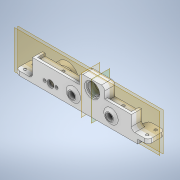
# Autodesk Inventor part: MotorBracket_v6.4
Saved by Autodesk Inventor 2022 (Build 260153000, 153)
## iProperties
Created: 2022-01-31
Part Number: MotorBracket_v6.4
Material: ABS プラスチック
Document SubType Name: Modeling
Designer: shiokaze
Density: 1.06 g/cm^3
Appearance: 滑らか - 白
Mass: 5.74152 g
Surface Area: 41.0545 cm^2
Volume: 5.41653 cm^3
Author: shiokaze
Autodesk Inventor part; units mm, degrees
ref_plane "YZ Plane" through (0, 0, 0) normal (1, 0, 0) x (0, 1, 0)
ref_plane "XZ Plane" through (0, 0, 0) normal (0, 1, 0) x (-1, 0, 0)
ref_plane "XY Plane" through (0, 0, 0) normal (0, 0, 1) x (1, 0, 0)
sketch "スケッチ2" plane through (0, 0, 0) normal (0, 0, 1) x (1, 0, 0)
  line L0 (-46.5, 9.7) -> (31.5, 9.7)
  line L1 (31.5, 9.7) -> (31.5, -9.7)
  line L2 (31.5, -9.7) -> (-46.5, -9.7)
  line L3 (-46.5, -9.7) -> (-46.5, 9.7)
  line L4 (-46.5, 9.7) -> (31.5, -9.7)
  line L5 (31.5, 9.7) -> (-46.5, -9.7)
  line L6 (-46.5, 9.7) -> (-8.95, 9.7)
  line L7 (-8.95, 9.7) -> (-8.95, -7.2)
  line L8 (-8.95, -7.2) -> (-46.5, -7.2)
  line L9 (-46.5, -7.2) -> (-46.5, 9.7)
  line L10 (31.5, 9.7) -> (5.95, 9.7)
  line L11 (5.95, 9.7) -> (5.95, -4.7)
  line L12 (5.95, -4.7) -> (31.5, -4.7)
  line L13 (31.5, -4.7) -> (31.5, 9.7)
  line L14 (-36.4485, -7.2) -> (-36.7, -7.2)
  line L15 (-36.7, -7.2) -> (-36.7, 3.5)
  line L16 (-36.7, 3.5) -> (-8.95, 3.5)
  line L17 (-8.95, 3.5) -> (-8.95, -0.3606)
  line L18 (5.95, -4.7) -> (21.7, -4.7)
  line L19 (21.7, -4.7) -> (21.7, 3.5)
  line L20 (21.7, 3.5) -> (5.95, 3.5)
  line L21 (5.95, 3.5) -> (5.95, -4.7)
  line L22 (31.5, -9.7) -> (25.5, -9.7)
  line L23 (25.5, -9.7) -> (25.5, -7.2)
  line L24 (25.5, -7.2) -> (31.5, -7.2)
  line L25 (31.5, -7.2) -> (31.5, -9.7)
  line L26 (-7.5, 0) -> (0, 0)
  point P0 (-7.5, 0)
  point P1 (5.95, 9.7)
  point P2 (-8.95, 9.7)
  point P3 (-8.95, 3.5)
  point P4 (-36.7, -7.2)
  point P5 (-46.5, -7.2)
  point P6 (31.5, -7.2)
  point P7 (31.5, -4.7)
  point P8 (21.7, -4.7)
  dimension "d0" = 78
  dimension "d1" = 19.4
  dimension "d15" = 37.55
  dimension "d16" = 2.5
  dimension "d17" = 25.55
  dimension "d18" = 6
  dimension "d19" = 2.5
  dimension "d20" = 9.8
  dimension "d21" = 9.8
  dimension "d26" = 7.5
  dimension "d188" = 10.7
  dimension "d241" = 5
  constraints: 54 end point, 12 parallel, 7 horizontal, 6 perpendicular, 3 collinear, 2 midpoint, 2 point on line, 1 coincident
  measures "d0" distance of L0.start L0.end
  measures "d1" distance of L0.end L1.end
  measures "d15" distance of L7.end L8.end
  measures "d16" distance between parallel lines of L2 L8
  measures "d17" distance of L12.end L11.end
  measures "d18" distance of L23.end L24.end
  measures "d19" distance of L22.end L23.end
  measures "d20" distance between parallel lines of L1 L19
  measures "d21" distance between parallel lines of L3 L15
  measures "d26" distance of L26.start L26.end
  measures "d188" distance between parallel lines of L16 L8
  measures "d241" distance between parallel lines of L18 L2
extrude "押し出し1" add sketch "スケッチ2" along normal blind 6 contours L0 L11 L5 L4 L7 | L8 L5 L3 | L16 L7 L4 | L4 L7 L5 L8 L15 L16 | L5 L8 L7 L4 L11 L12 L23 L2 | L4 L5 L7 | L20 L5 L11 | L5 L7 L8 | L5 L11 L4 | L1 L24 L23 L4 L12 | L20 L19 L12 L4 L11 L5 | L4 L12 L11
sketch "スケッチ8" plane through (0, 0, 6) normal (0, 0, 1) x (1, 0, 0)
  circle A0 centre (-1.5, 4.4354) radius 3.85 construction
  circle A1 centre (9.625, -3.3) radius 9.7 construction
  circle A2 centre (-12.625, -3.3) radius 9.7 construction
  circle A3 centre (-26.1025, -4.7) radius 3.85 construction
  line L0 (-46.5, -9.7) -> (25.5, -9.7) construction
  circle A4 centre (-12.625, -3.3) radius 10.5
  circle A5 centre (9.625, -3.3) radius 10.5
  line L1 (-2.125, -3.3) -> (-0.875, -3.3)
  line L2 (-12.625, -3.3) -> (-1.5, 4.4354) construction
  line L3 (-1.5, 4.4354) -> (9.625, -3.3) construction
  line L4 (-26.1025, -4.7) -> (-12.625, -3.3) construction
  line L5 (-46.5, -9.7) -> (25.5, -9.7) projected
  line L6 (-46.5, -9.7) -> (25.5, -9.7)
  line L7 (25.5, -9.7) -> (25.5, -11.3)
  line L8 (25.5, -11.3) -> (-46.5, -11.3) construction
  line L9 (-46.5, -11.3) -> (-46.5, -9.7)
  line L10 (-46.5, -11.3) -> (25.5, -11.3)
  line L11 (25.5, -11.3) -> (25.5, -13.8)
  line L12 (25.5, -13.8) -> (-46.5, -13.8) construction
  line L13 (-46.5, -13.8) -> (-46.5, -11.3)
  line L14 (25.5, -9.7) -> (25.5, -7.2) projected
  line L15 (5.95, 9.7) -> (-8.95, 9.7) projected
  circle A6 centre (-26.1025, -4.7) radius 5
  point P0 (0, 0)
  point P1 (-1.5, 9.7)
  dimension "d123" = 21
  dimension "d124" = 21
  dimension "d29" = 7.7
  dimension "d30" = 19.4
  dimension "d31" = 19.4
  dimension "d32" = 7.7
  dimension "d132" = 1.25
  dimension "d147" = 1.6
  dimension "d148" = 2.5
  dimension "d164" = 10
  constraints: 24 end point, 7 coincident, 5 centre point, 4 horizontal, 4 parallel, 2 collinear, 2 equal length, 2 horizontal alignment, 2 perpendicular, 2 point on line, 2 tangent, 1 midpoint, 1 vertical alignment, 4 other
  measures "d29" diameter of A0
  measures "d30" diameter of A2
  measures "d31" diameter of A1
  measures "d32" diameter of A3
  measures "d132" distance of L1.start L1.end
  measures "d147" distance of L6.end L7.end
  measures "d148" distance of L10.end L11.end
  measures "d164" diameter of A6
hole "穴1" at (-12.625, -3.3, 6) at (9.625, -3.3, 6) at (-1.5, 4.4354, 6) at (-26.1025, -4.7, 6) direction (0, 0, -1) diameter 0.1 end through all
sketch "スケッチ22" plane through (0, 0, 6) normal (0, 0, 1) x (1, 0, 0)
  circle A0 centre (9.625, -3.3) radius 0.05 projected
  circle A1 centre (-12.625, -3.3) radius 0.05 projected
  circle A2 centre (-26.1025, -4.7) radius 0.05 projected
  point P0 (0, 0)
  constraints: 3 coincident
hole "穴8" at (-12.625, -3.3, 6) at (9.625, -3.3, 6) direction (0, 0, -1) diameter 4 end through all
sketch "スケッチ23" plane through (0, 0, 6) normal (0, 0, 1) x (1, 0, 0)
  circle A0 centre (-1.5, 4.4354) radius 0.05 projected
  point P0 (0, 0)
  constraints: 1 coincident
hole "穴9" at (-1.5, 4.4354, 6) direction (0, 0, -1) diameter 7 end through all
sketch "スケッチ27" plane through (0, 0, 6) normal (0, 0, 1) x (1, 0, 0)
  circle A0 centre (-26.1025, -4.7) radius 0.05 projected
  point P0 (0, 0)
  constraints: 1 coincident
hole "穴10" at (-26.1025, -4.7, 6) direction (0, 0, -1) diameter 10.1 end through all
sketch "スケッチ28" plane through (0, 0, 6) normal (0, 0, 1) x (1, 0, 0)
  circle A0 centre (-26.0019, -4.7) radius 2
  arc A1 (-25.3936, -9.7) -> (-26.8114, -9.7) centre (-26.1025, -4.7) ccw projected
  arc A2 (-25.3936, -9.7) -> (-26.8114, -9.7) centre (-26.1025, -4.7) ccw projected
  line L0 (-25.3936, -9.7) -> (-26.8114, -9.7)
  point P0 (0, 0)
  point P1 (-26.8114, -9.7)
  dimension "d173" = 4
  constraints: 2 end point, 1 centre point, 1 coincident, 1 horizontal, 1 point on circle
  measures "d173" diameter of A0
extrude "押し出し8" add sketch "スケッチ28" against normal blind 1.5
sketch "スケッチ29" plane through (-26.1025, -4.7, 4.5) normal (0, 0, -1) x (1, 0, 0)
  circle A0 centre (0.1005, 0) radius 2 projected
  point P0 (26.1025, -4.7)
  point P1 (-3.3995, 0)
  point P2 (0.1005, 3.5)
  point P3 (3.6005, 0)
  point P4 (0.1005, -3.5)
  dimension "d176" = 3.5
  dimension "d179" = 360
  constraints: 1 coincident, 1 horizontal alignment, 5 other
  measures "d176" distance of point (0.101, 0) point (-3.399, 0)
hole "穴11" at (-29.5019, -4.7, 4.5) at (-26.0019, -4.7, 4.5) at (-22.5019, -4.7, 4.5) direction (0, 0, 1) diameter 1.8 end through all
sketch "スケッチ30" plane through (0, 0, 0) normal (0, 0, -1) x (-1, 0, 0)
  circle A0 centre (1.5, 4.4354) radius 3.5 projected
  circle A1 centre (1.5, 4.4354) radius 4.5
  point P0 (0, 0)
  dimension "d189" = 9
  constraints: 1 centre point, 1 coincident
  measures "d189" diameter of A1
extrude "押し出し9" cut sketch "スケッチ30" against normal blind 1
sketch "スケッチ31" plane through (-46.5, -9.7, 6) normal (0, -1, 0) x (1, 0, 0)
  line L0 (49.5, -7.5) -> (40.5, -7.5)
  line L1 (40.5, -7.5) -> (40.5, -2.5)
  line L2 (40.5, -2.5) -> (49.5, -2.5)
  line L3 (49.5, -2.5) -> (49.5, -7.5)
  line L4 (49.5, -6) -> (40.5, -6) projected
  line L5 (49.5, -5) -> (40.5, -5) projected
  line L6 (49.5, -6) -> (40.5, -6) projected
  line L7 (0, 0) -> (72, 0) projected
  line L8 (55, -1.6369) -> (35, -1.6369)
  line L9 (35, -1.6369) -> (35, -10)
  line L10 (35, -10) -> (55, -10)
  line L11 (55, -10) -> (55, -1.6369)
  point P0 (46.5, -6)
  point P1 (45, -10)
  point P2 (45, -7.5)
  dimension "d192" = 5
  dimension "d193" = 7.5
  dimension "d194" = 10
  dimension "d195" = 20
  constraints: 16 end point, 4 midpoint, 4 parallel, 2 horizontal, 2 perpendicular, 1 vertical alignment
  measures "d192" distance between parallel lines of L0 L2
  measures "d193" distance between parallel lines of L0 L7
  measures "d194" distance between parallel lines of L10 L7
  measures "d195" distance of L9.end L10.end
extrude "押し出し10" add sketch "スケッチ31" against normal blind 1.5
sketch "スケッチ32" plane through (-46.5, -9.7, 6) normal (0, -1, 0) x (1, 0, 0)
  line L0 (52.5, -7.5) -> (37.5, -7.5)
  line L1 (52.5, -7.5) -> (37.5, -7.5)
  line L2 (37.5, -7.5) -> (37.5, -2.5)
  line L3 (37.5, -2.5) -> (52.5, -2.5)
  line L4 (52.5, -2.5) -> (52.5, -7.5)
  line L5 (37.5, -7.5) -> (37.5, -6)
  line L6 (41.5, -5) -> (48.5, -5) projected
  line L7 (0, 0) -> (72, 0) projected
  point P0 (45, -2.5)
  point P1 (45, -5)
  dimension "d198" = 5
  dimension "d204" = 15
  dimension "d205" = 2.5
  constraints: 12 end point, 2 midpoint, 2 parallel, 1 collinear, 1 horizontal, 1 perpendicular, 1 vertical alignment
  measures "d198" distance of L1.end L2.end
  measures "d204" distance between parallel lines of L4 L2
  measures "d205" distance between parallel lines of L3 L7
extrude "押し出し11" add sketch "スケッチ32" along normal blind 1.6
sketch "スケッチ33" plane through (-46.5, -9.7, 6) normal (0, 1, 0) x (1, 0, 0)
  line L0 (52.5, 2.5) -> (37.5, 2.5) projected
  line L1 (37.5, 2.5) -> (37.5, 7.5) projected
  line L2 (37.5, 7.5) -> (52.5, 7.5) projected
  line L3 (52.5, 7.5) -> (52.5, 2.5) projected
extrude "押し出し12" add sketch "スケッチ33" along normal up to surface (1.5 mm away)
fillet "フィレット14" radius 2 4 edges at (6, -10.5, -1.5) (6, -10.5, 3.5) (-9, -10.5, -1.5) (-9, -10.5, 3.5)
sketch "スケッチ34" plane through (0, 0, 0) normal (0, 0, -1) x (-1, 0, 0)
  line L0 (-31.5, -4.7) -> (-21.7, -4.7) projected
  line L1 (-31.5, -7.2) -> (-31.5, -4.7) projected
  line L2 (-25.5, -7.2) -> (-31.5, -7.2) projected
  line L3 (-8.5, -9.7) -> (-25.5, -9.7) projected
  line L4 (-25.5, -9.7) -> (-25.5, -7.2) projected
  line L5 (-21.7, -4.7) -> (-21.7, 3.5) projected
  line L6 (36.7, -7.2) -> (46.5, -7.2) projected
  line L7 (36.7, 3.5) -> (36.7, -7.2) projected
  line L8 (46.5, -9.7) -> (26.8114, -9.7) projected
  line L9 (46.5, -7.2) -> (46.5, -9.7) projected
  line L10 (-31.5, -4.7) -> (-21.7, -4.7)
  line L11 (-21.7, -4.7) -> (-21.7, -7.2)
  line L12 (-21.7, -7.2) -> (-31.5, -7.2)
  line L13 (-31.5, -7.2) -> (-31.5, -4.7)
  line L14 (46.5, -9.7) -> (-25.5, -9.7) projected
  line L15 (-21.7, -9.7) -> (-25.5, -9.7)
  line L16 (-25.5, -9.7) -> (-25.5, -7.2)
  line L17 (-25.5, -7.2) -> (-21.7, -7.2)
  line L18 (-21.7, -7.2) -> (-21.7, -9.7)
  line L19 (36.7, -7.2) -> (46.5, -7.2)
  line L20 (46.5, -7.2) -> (46.5, -9.7)
  line L21 (46.5, -9.7) -> (36.7, -9.7)
  line L22 (36.7, -9.7) -> (36.7, -7.2)
  point P0 (0, 0)
  point P1 (26.0019, -9.7)
  point P2 (36.7, -9.7)
  point P3 (-21.7, -4.7)
  constraints: 24 end point, 6 parallel, 3 horizontal, 3 perpendicular, 2 collinear, 2 point on line
extrude "押し出し13" add sketch "スケッチ34" along normal blind 10 from surface at -6
fillet "フィレット15" radius 2 8 edges at (21.7, -7.2, -4) (21.7, -7.2, 0) (-36.7, -8.45, 0) (-36.7, -8.45, -4) (31.5, -5.95, -4) (31.5, -5.95, 6) (-46.5, -8.45, -4) (-46.5, -8.45, 6)
fillet "フィレット16" radius 2 2 edges at (21.7, -4.7, 3) (-36.7, -7.2, 3)
fillet "フィレット17" radius 1.5 5 edges at (8.5, -8.95, -4) (-11.5, -8.95, -4) (-1.5, -8.2, 0) (8.5, -8.95, 0) (-11.5, -8.95, 0)
sketch "スケッチ35" plane through (-36.7, 3.5, 0) normal (0, 1, 0) x (1, 0, 0)
  line L0 (27.75, 0) -> (0, 0) projected
  line L1 (0, 0) -> (0, -6) projected
  line L2 (27.75, -6) -> (0, -6) projected
  line L3 (27.75, 0) -> (27.75, -6) projected
  line L4 (58.4, 0) -> (42.65, 0) projected
  line L5 (42.65, 0) -> (42.65, -6) projected
  line L6 (58.4, -6) -> (42.65, -6) projected
  line L7 (58.4, 0) -> (58.4, -6) projected
  line L8 (27.75, 0) -> (1.5, 0)
  line L9 (1.5, 0) -> (1.5, -4.5)
  line L10 (1.5, -4.5) -> (27.75, -4.5)
  line L11 (27.75, -4.5) -> (27.75, 0)
  line L12 (42.65, 0) -> (56.9, 0)
  line L13 (56.9, 0) -> (56.9, -4.5)
  line L14 (56.9, -4.5) -> (42.65, -4.5)
  line L15 (42.65, -4.5) -> (42.65, 0)
  point P0 (36.7, 0)
  point P1 (1.5, 0)
  dimension "d277" = 1.5
  dimension "d278" = 1.5
  dimension "d279" = 1.5
  dimension "d280" = 1.5
  constraints: 16 end point, 4 parallel, 2 horizontal, 2 perpendicular, 1 coincident
  measures "d277" distance between parallel lines of L7 L13
  measures "d278" distance between parallel lines of L1 L9
  measures "d279" distance between parallel lines of L6 L14
  measures "d280" distance between parallel lines of L2 L10
extrude "押し出し14" cut sketch "スケッチ35" against normal blind 1.6 contours L3 L10 L9 L0 | L13 L14 L5 L4
sketch "スケッチ37" plane through (-36.7, 1.9, 0) normal (0, 1, 0) x (1, 0, 0)
  line L0 (27.75, 0) -> (27.75, -6) projected
  line L1 (1.5, 0) -> (27.75, 0) projected
  line L2 (42.65, 0) -> (42.65, -6) projected
  line L3 (56.9, 0) -> (56.9, -4.5) projected
  line L4 (1.5, -4.5) -> (1.5, 0) projected
  point P0 (36.7, 0)
  point P1 (14.45, -2.25)
  point P2 (49.95, -2.25)
  dimension "d220" = 2.25
  dimension "d264" = 6.95
  dimension "d265" = 12.95
  constraints: 1 horizontal alignment
  measures "d220" distance from line of L1 point (14.45, -2.25)
  measures "d264" distance from line of L3 point (49.95, -2.25)
  measures "d265" distance from line of L4 point (14.45, -2.25)
hole "穴12" at (-22.25, 1.9, 2.25) at (13.25, 1.9, 2.25) direction (0, -1, 0) diameter 1.567 depth 0.1 tip angle 118 thread size "M2x0.4" class "6H" standard "ISO Metric profile"
ref_plane "作業平面3" through (-7.5, -7.2, 4) normal (1, 0, 0) x (0, 0, -1)
ref_plane "作業平面4" through (-1.5, 3.5, 6) normal (-1, 0, 0) x (0, 0, 1)
ref_plane "作業平面5" through (-7, -9.7, 1) normal (0, 0, 1) x (1, 0, 0)
ref_plane "作業平面6" through (0, 0, 3) normal (0, 0, 1) x (1, 0, 0)
sketch "スケッチ40" plane through (23.7, -4.7, -4) normal (0, 1, 0) x (1, 0, 0)
  line L0 (7.8, -10) -> (4.8, -10)
  line L1 (4.8, -10) -> (4.8, -7.5)
  line L2 (4.8, -7.5) -> (7.8, -7.5)
  line L3 (7.8, -7.5) -> (7.8, -10)
  line L4 (5.8, -10) -> (0, -10) projected
  line L5 (7.8, -2) -> (7.8, -8) projected
  point P0 (-23.7, -4)
  dimension "d231" = 3
  dimension "d232" = 2.5
  constraints: 8 end point, 2 collinear, 2 parallel, 1 coincident, 1 horizontal, 1 perpendicular
  measures "d231" distance of L1.end L2.end
  measures "d232" distance of L0.end L1.end
hole "穴13" at (28.5, -4.7, 3.5) direction (0, -1, 0) diameter 1.567 depth 0.1 tip angle 118 thread size "M2x0.4" class "6H" standard "ISO Metric profile"
mirror "ミラー2" about plane through (-7, -9.7, 1) normal (0, 0, 1) of "穴13"
fillet "フィレット18" radius 2 2 edges at (5.95, 9.7, 3) (-8.95, 9.7, 3)
sketch "スケッチ42" plane through (-44.5, -7.2, -4) normal (0, 1, 0) x (1, 0, 0)
  line L0 (5.8, -10) -> (0, -10) projected
  line L1 (-2, -2) -> (-2, -8) projected
  line L2 (-2, -10) -> (1, -10)
  line L3 (1, -10) -> (1, -7.5)
  line L4 (1, -7.5) -> (-2, -7.5)
  line L5 (-2, -7.5) -> (-2, -10)
  point P0 (44.5, -4)
  dimension "d242" = 3
  dimension "d243" = 2.5
  constraints: 8 end point, 2 parallel, 1 coincident, 1 collinear, 1 horizontal, 1 perpendicular, 1 point on line
  measures "d242" distance of L4.end L3.end
  measures "d243" distance of L3.end L2.end
hole "穴14" at (-43.5, -7.2, 3.5) direction (0, -1, 0) diameter 1.567 depth 0.1 tip angle 118 thread size "M2x0.4" class "6H" standard "ISO Metric profile"
mirror "ミラー4" about plane through (-7, -9.7, 1) normal (0, 0, 1) of "穴14"
sketch "スケッチ43" plane through (0, 0, 6) normal (0, 0, 1) x (1, 0, 0)
  circle A0 centre (9.625, -3.3) radius 2 projected
  circle A1 centre (9.625, -3.3) radius 2.5
  circle A2 centre (-12.625, -3.3) radius 2 projected
  circle A3 centre (-12.625, -3.3) radius 2.5
  point P0 (0, 0)
  dimension "d251" = 5
  dimension "d252" = 5
  constraints: 2 centre point, 2 coincident
  measures "d251" diameter of A1
  measures "d252" diameter of A3
extrude "押し出し15" add sketch "スケッチ43" along normal blind 1
fillet "フィレット19" radius 2 2 edges at (7.125, -3.3, 6) (-15.125, -3.3, 6)
sketch "スケッチ44" plane through (0, 0, 6) normal (0, 0, 1) x (1, 0, 0)
  circle A0 centre (-1.5, 4.4354) radius 4.5 projected
  point P0 (0, 0)
extrude "押し出し16" cut sketch "スケッチ44" against normal blind 1
chamfer "面取り1" distance 0.2 angle 45 2 edges at (-1.5, 7.9354, 1) (-1.5, 7.9354, 5)
sketch "スケッチ45" plane through (0, 0, 0) normal (0, 0, -1) x (-1, 0, 0)
  arc A0 (26.8114, -9.7) -> (25.3936, -9.7) centre (26.1025, -4.7) ccw projected
  arc A1 (30.4106, -9.7) -> (21.7943, -9.7) centre (26.1025, -4.7) ccw
  line L0 (44.5, -9.7) -> (-25.5, -9.7) projected
  line L1 (25.3936, -9.7) -> (13, -9.7) projected
  line L2 (35.2, 1.9) -> (8.95, 1.9) projected
  line L3 (34.7, -9.7) -> (13, -9.7) projected
  point P0 (0, 0)
  point P1 (26.0019, -9.7)
  point P2 (21.7943, -9.7)
  point P3 (30.4106, -9.7)
  point P4 (26.8114, -9.7)
  constraints: 2 point on circle, 2 point on line, 1 centre point, 1 coincident, 1 tangent, 1 other
extrude "押し出し17" add sketch "スケッチ45" along normal up to surface (4 mm away) contours A0 L0 A1
fillet "フィレット20" radius 2 2 edges at (-19.9154, -2.4022, 0) (-32.2896, -2.4022, 0)
sketch "スケッチ49" plane through (0, 0, 0) normal (0, 0, -1) x (-1, 0, 0)
  line L0 (-2.4299, -2.531) -> (5.5013, -2.531) construction
  line L1 (5.5013, -2.531) -> (5.5013, -5.7001) construction
  line L2 (5.5013, -5.7001) -> (-2.4299, -5.7001) construction
  line L3 (-2.4299, -5.7001) -> (-2.4299, -2.531) construction
  line L4 (-0.3551, -3.3486) -> (-1.2171, -5.6359)
  line L5 (-1.2171, -5.6359) -> (-1.5629, -5.6359)
  line L6 (-1.5629, -5.6359) -> (-2.4175, -3.3486)
  line L7 (-2.4175, -3.3486) -> (-2.0001, -3.3486)
  line L8 (-2.0001, -3.3486) -> (-1.3752, -5.1097)
  line L9 (-1.3752, -5.1097) -> (-0.7552, -3.3486)
  line L10 (-0.7552, -3.3486) -> (-0.3551, -3.3486)
  spline S0 degree 2 poles (1.8062, -4.6478) (1.8062, -4.8825) (1.6506, -5.2802) (1.5197, -5.4136) knots 0 0 0 1 2 2 2
  spline S1 degree 2 poles (1.5197, -5.4136) (1.3838, -5.5543) (1.043, -5.7001) (0.8379, -5.7001) knots 0 0 0 1 2 2 2
  spline S2 degree 2 poles (0.8379, -5.7001) (0.6329, -5.7001) (0.2945, -5.5618) (0.1661, -5.4234) knots 0 0 0 1 2 2 2
  spline S3 degree 2 poles (0.1661, -5.4234) (0.008, -5.2579) (-0.1698, -4.7022) (-0.1698, -4.2971) knots 0 0 0 1 2 2 2
  spline S4 degree 2 poles (-0.1698, -4.2971) (-0.1698, -3.8994) (-0.0068, -3.2597) (0.1636, -3.0226) knots 0 0 0 1 2 2 2
  spline S5 degree 2 poles (0.1636, -3.0226) (0.3291, -2.7904) (0.8528, -2.531) (1.1961, -2.531) knots 0 0 0 1 2 2 2
  spline S6 degree 2 poles (1.1961, -2.531) (1.2974, -2.531) (1.4752, -2.5508) (1.5419, -2.573) knots 0 0 0 1 2 2 2
  line L11 (1.5419, -2.573) -> (1.5419, -2.9658)
  line L12 (1.5419, -2.9658) -> (1.5246, -2.9658)
  spline S7 degree 2 poles (1.5246, -2.9658) (1.4678, -2.9361) (1.2603, -2.8843) (1.1418, -2.8843) knots 0 0 0 1 2 2 2
  spline S8 degree 2 poles (1.1418, -2.8843) (0.7614, -2.8843) (0.2945, -3.398) (0.2501, -3.9019) knots 0 0 0 1 2 2 2
  spline S9 degree 2 poles (0.2501, -3.9019) (0.3958, -3.8006) (0.7021, -3.6895) (0.8849, -3.6895) knots 0 0 0 1 2 2 2
  spline S10 degree 2 poles (0.8849, -3.6895) (1.0627, -3.6895) (1.3295, -3.7611) (1.4752, -3.8698) knots 0 0 0 1 2 2 2
  spline S11 degree 2 poles (1.4752, -3.8698) (1.6432, -3.9958) (1.8062, -4.386) (1.8062, -4.6478) knots 0 0 0 1 2 2 2
  spline S12 degree 2 poles (1.3912, -4.6651) (1.3912, -4.4774) (1.2924, -4.223) (1.1837, -4.1341) knots 0 0 0 1 2 2 2
  spline S13 degree 2 poles (1.1837, -4.1341) (1.1022, -4.0699) (0.8997, -4.0279) (0.7935, -4.0279) knots 0 0 0 1 2 2 2
  spline S14 degree 2 poles (0.7935, -4.0279) (0.6502, -4.0279) (0.381, -4.1143) (0.2501, -4.1958) knots 0 0 0 1 2 2 2
  spline S15 degree 2 poles (0.2501, -4.1958) (0.2476, -4.2403) (0.2427, -4.3243) (0.2427, -4.3885) knots 0 0 0 1 2 2 2
  spline S16 degree 2 poles (0.2427, -4.3885) (0.2427, -4.7047) (0.3662, -5.0924) (0.46, -5.1937) knots 0 0 0 1 2 2 2
  spline S17 degree 2 poles (0.46, -5.1937) (0.5465, -5.29) (0.7342, -5.3666) (0.8404, -5.3666) knots 0 0 0 1 2 2 2
  spline S18 degree 2 poles (0.8404, -5.3666) (1.0874, -5.3666) (1.3912, -5.0159) (1.3912, -4.6651) knots 0 0 0 1 2 2 2
  line L13 (2.8214, -5.6359) -> (2.3323, -5.6359)
  line L14 (2.3323, -5.6359) -> (2.3323, -5.0529)
  line L15 (2.3323, -5.0529) -> (2.8214, -5.0529)
  line L16 (2.8214, -5.0529) -> (2.8214, -5.6359)
  line L17 (5.3976, -4.5886) -> (5.0345, -4.5886)
  line L18 (5.0345, -4.5886) -> (5.0345, -5.6359)
  line L19 (5.0345, -5.6359) -> (4.6418, -5.6359)
  line L20 (4.6418, -5.6359) -> (4.6418, -4.5886)
  line L21 (4.6418, -4.5886) -> (3.2956, -4.5886)
  line L22 (3.2956, -4.5886) -> (3.2956, -4.1588)
  line L23 (3.2956, -4.1588) -> (4.6591, -2.5879)
  line L24 (4.6591, -2.5879) -> (5.0345, -2.5879)
  line L25 (5.0345, -2.5879) -> (5.0345, -4.2601)
  line L26 (5.0345, -4.2601) -> (5.3976, -4.2601)
  line L27 (5.3976, -4.2601) -> (5.3976, -4.5886)
  line L28 (4.6418, -4.2601) -> (4.6418, -3.0695)
  line L29 (4.6418, -3.0695) -> (3.6167, -4.2601)
  line L30 (3.6167, -4.2601) -> (4.6418, -4.2601)
  point P0 (0, 0)
  constraints: 2 other
extrude "押し出し19" cut sketch "スケッチ49" against normal blind 0.25
